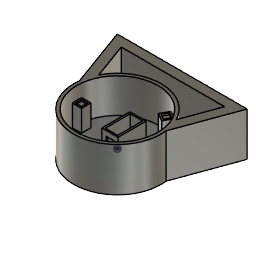
base (Autodesk Fusion 360 design; units mm, degrees)
part number: 2026-04-11-20-46-35-082
Autodesk Fusion 360 part; units mm, degrees
note: some values were not read from the file. Chosen so that the rebuilt part matches the saved one: which bodies a step acts on; that a step has no effect; which face or edge a step refers to. Set by a fixed rule: which sketch regions a step uses.
sketch "Esboço1" plane through (0, 0, 0) normal (0, 0, 1) x (1, 0, 0)
  circle A0 centre (0, 0) radius 70
  circle A1 centre (0, 0) radius 65
  dimension "d1" = 140
  dimension "d2" = 130
  constraint coincident A0.centre A1.centre
  measures "d1" diameter of A0
  measures "d2" diameter of A1
extrude "Extrusão1" add sketch "Esboço1" along normal blind 45 makes body 1
sketch "Esboço2" plane through (0, 0, 0) normal (0, 0, 1) x (1, 0, 0)
  circle A0 centre (0, 0) radius 70
  constraint coincident A0.centre origin
extrude "Extrusão2" add sketch "Esboço2" along normal blind 5 bodies 1
sketch "Esboço3" plane through (0, 0, 0) normal (0, 0, 1) x (1, 0, 0)
  line L0 (-9.5, 19.5) -> (9.5, 19.5)
  line L1 (9.5, 19.5) -> (9.5, -19.5)
  line L2 (9.5, -19.5) -> (-9.5, -19.5)
  line L3 (-9.5, -19.5) -> (-9.5, 19.5)
  line L4 (-9.75, -19.75) -> (9.75, -19.75)
  line L5 (9.75, -19.75) -> (9.75, 19.75)
  line L6 (9.75, 19.75) -> (-9.75, 19.75)
  line L7 (-9.75, 19.75) -> (-9.75, -19.75)
  circle A0 centre (0, 0) radius 70
  line L8 (0, 0) -> (9.5, 0)
  line L9 (0, 0) -> (0, -19.5)
  dimension "d7" = 19
  dimension "d8" = 39
  dimension "d9" = 19.5
  dimension "d10" = 39.5
  dimension "d15" = 9.5
  dimension "d16" = 19.5
  constraint horizontal L0
  constraint vertical L1
  constraint horizontal L2
  constraint vertical L3
  constraint horizontal L4
  constraint vertical L5
  constraint horizontal L6
  constraint vertical L7
  constraint coincident A0.centre L8.start
  constraint perpendicular L5 L8
  constraint perpendicular L8 L9
  constraint coincident L2 L9.end
  constraint coincident L1 L8.end
  measures "d7" distance of L0.start L0.end
  measures "d8" distance of L0.start L2.end
  measures "d9" distance of L4.start L4.end
  measures "d10" distance of L4.start L6.end
  measures "d15" distance of A0.centre L8.end
  measures "d16" distance of A0.centre L9.end
sketch "Esboço5" plane through (0, 0, 0) normal (0, 0, 1) x (1, 0, 0)
sketch "Esboço6" plane through (0, 0, 0) normal (0, 0, -1) x (1, 0, 0)
  circle A0 centre (0, 0) radius 70
  line L0 (-9.5, 19.5) -> (9.5, 19.5)
  line L1 (9.5, 19.5) -> (9.5, -19.5)
  line L2 (9.5, -19.5) -> (-9.5, -19.5)
  line L3 (-9.5, -19.5) -> (-9.5, 19.5)
  line L4 (-70, 0) -> (70, 0)
  line L5 (-12, 22) -> (12, 22)
  line L6 (12, 22) -> (12, -22)
  line L7 (12, -22) -> (-12, -22)
  line L8 (-12, -22) -> (-12, 22)
  dimension "d19" = 19
  dimension "d20" = 39
  dimension "d21" = 24
  dimension "d22" = 44
  constraint horizontal L0
  constraint vertical L1
  constraint horizontal L2
  constraint vertical L3
  constraint coincident A0 L4.start
  constraint coincident A0 L4.end
  constraint horizontal L5
  constraint vertical L6
  constraint horizontal L7
  constraint vertical L8
  measures "d19" distance of L0.start L0.end
  measures "d20" distance of L0.start L2.end
  measures "d21" distance of L5.start L5.end
  measures "d22" distance of L5.start L7.end
extrude "Extrusão4" add sketch "Esboço6" against normal blind 38 contours L1 L2 L3 L4 L6 L7 L8 | L0 L1 L3 L4 L5 L6 L8 bodies 1
move_body "Mover1" bodies 1 to x (1, 0, 0) y (0, 1, 0) z (0, 0, 1) at (0, 0, 10)
extrude "Extrusão5" add 1 faces at (2.4201, -10.6031, 10) along direction (0, 0, -1) blind 10 on bodies 1 bodies 1
sketch "Esboço7" plane through (0, 0, 15) normal (0, 0, 1) x (-1, 0, 0)
  circle A0 centre (0, 0) radius 65
  line L0 (-12, -22) -> (-12, 22)
  line L1 (-12, 22) -> (12, 22)
  line L2 (12, 22) -> (12, -22)
  line L3 (12, -22) -> (-12, -22)
  line L4 (-20, 30) -> (20, 30)
  line L5 (20, 30) -> (20, -30)
  line L6 (20, -30) -> (-20, -30)
  line L7 (-20, -30) -> (-20, 30)
  constraint horizontal L4
  constraint vertical L5
  constraint horizontal L6
  constraint vertical L7
extrude "Extrusão6" cut sketch "Esboço7" along normal blind 0.01 contours L0 L1 L2 L3 | L4 L5 L6 L7 bodies 1 makes body 2 at (69.913, -3.4892, 18.3333)
sketch "Esboço8" plane through (0, 0, 15) normal (0, 0, 1) x (-1, 0, 0)
  circle A0 centre (0, 0) radius 65
  circle A1 centre (0, 0) radius 2.5
  dimension "d29" = 5
  constraint coincident A0.centre A1.centre
  measures "d29" diameter of A1
move_body "Mover2" bodies 1 to x (1, 0, 0) y (0, 1, 0) z (0, 0, 1) at (0, 9, 0)
move_body "Mover3" bodies 1 to x (1, 0, 0) y (0, 1, 0) z (0, 0, 1) at (0, 1.5, 0)
move_body "Mover4" bodies 1 to x (1, 0, 0) y (0, 1, 0) z (0, 0, 1) at (0, 0, -0.02)
combine "Combinar1" operation add target body 2 tool bodies 1
fillet "Arredondamento1" radius 5 tangency weight 0.69913 4 edges at (-12, 10.5, 15) (0, -11.5, 15) (12, 10.5, 15) (0, 32.5, 15) on bodies 2
sketch "Esboço9" plane through (0, -11.5, 0) normal (0, -1, 0) x (1, 0, 0)
  line L0 (12, 20) -> (-12, 20)
  line L1 (12, 20) -> (12, 47.98)
  line L2 (12, 47.98) -> (-12, 47.98)
  line L3 (-12, 47.98) -> (-12, 20)
  line L4 (-4.8756, 37.7433) -> (5.1244, 37.7433)
  line L5 (5.1244, 37.7433) -> (5.1244, 22.7433)
  line L6 (5.1244, 22.7433) -> (-4.8756, 22.7433)
  line L7 (-4.8756, 22.7433) -> (-4.8756, 37.7433)
  dimension "d32" = 10
  dimension "d33" = 15
  constraint horizontal L4
  constraint vertical L5
  constraint horizontal L6
  constraint vertical L7
  measures "d32" distance of L4.start L4.end
  measures "d33" distance of L4.start L6.end
extrude "Extrusão7" add sketch "Esboço9" along normal blind 22 separate body contours L4 L5 L6 L7 makes body 3
move_body "Mover5" bodies 3 to x (1, 0, 0) y (0, 1, 0) z (0, 0, 1) at (0, 0, -7.743)
move_body "Mover6" bodies 3 to x (1, 0, 0) y (0, 1, 0) z (0, 0, 1) at (-0.124, 0, 0)
move_body "Mover7" bodies 3 to x (1, 0, 0) y (0, 1, 0) z (0, 0, 1) at (0, 60, 0)
combine "Combinar2" operation cut target body 2 tool bodies 3
extrude "Extrusão8" cut 1 faces at (-11.1667, 4, 47.98) along direction (0, 0, -1) blind 4.98 on bodies 2 bodies 2
sketch "Esboço10" plane through (0, 0, 15) normal (0, 0, 1) x (-1, 0, 0)
  line L0 (-32.5, 56.2917) -> (-26.0048, 60.0417)
  line L1 (-32.5, 56.2917) -> (-38.9952, 52.5417)
  line L2 (-38.9952, 52.5417) -> (-30.9952, 38.6852)
  line L3 (-26.0048, 60.0417) -> (-18.5048, 47.0513)
  line L4 (-18.5048, 47.0513) -> (-31.4952, 39.5513)
  line L5 (-32.5, -56.2917) -> (-38.9952, -52.5417)
  line L6 (-32.5, -56.2917) -> (-26.0048, -60.0417)
  line L7 (-38.9952, -52.5417) -> (-31.4952, -39.5513)
  line L8 (-26.0048, -60.0417) -> (-18.5048, -47.0513)
  line L9 (-31.4952, -39.5513) -> (-18.5048, -47.0513)
  line L10 (65, 0) -> (65, 7.5)
  line L11 (65, 0) -> (65, -7.5)
  line L12 (65, 7.5) -> (50, 7.5)
  line L13 (65, -7.5) -> (50, -7.5)
  line L14 (50, 7.5) -> (50, -7.5)
  line L15 (59.9632, 5) -> (62.5, 5)
  line L16 (52.5, 1) -> (52.5, -5)
  line L17 (52.5, 5) -> (52.5, 1)
  line L18 (52.5, -5) -> (62.5, -5)
  line L19 (62.5, 5) -> (62.5, -5)
  line L20 (52.5, 5) -> (62.5, 5)
  line L21 (-24.9107, -53.1467) -> (-26.9199, -56.6266)
  line L22 (-33.0801, -47.2965) -> (-30.5801, -42.9663)
  line L23 (-31.25, -54.1266) -> (-35.5801, -51.6266)
  line L24 (-24.9107, -53.1467) -> (-21.9199, -47.9663)
  line L25 (-35.5801, -51.6266) -> (-26.9199, -56.6266)
  line L26 (-35.5801, -51.6266) -> (-30.5801, -42.9663)
  line L27 (-30.5801, -42.9663) -> (-21.9199, -47.9663)
  line L28 (-21.9199, -47.9663) -> (-26.9199, -56.6266)
  line L29 (-31.25, 54.1266) -> (-35.5801, 51.6266)
  line L30 (-24.4199, 52.2965) -> (-26.9199, 56.6266)
  line L31 (-26.25, 45.4663) -> (-21.9199, 47.9663)
  line L32 (-30.5801, 42.9663) -> (-21.9199, 47.9663)
  line L33 (-21.9199, 47.9663) -> (-26.9199, 56.6266)
  line L34 (-26.9199, 56.6266) -> (-35.5801, 51.6266)
  line L35 (-35.5801, 51.6266) -> (-30.5801, 42.9663)
  dimension "d39" = 65
  dimension "d41" = 7.5
  dimension "d42" = 7.5
  dimension "d43" = 16
  dimension "d44" = 15
  dimension "d52" = 7.5
  dimension "d53" = 7.5
  dimension "d54" = 15
  dimension "d55" = 15
  dimension "d57" = 7.5
  dimension "d58" = 7.5
  dimension "d59" = 15
  dimension "d60" = 15
  dimension "d64" = 2.5
  dimension "d68" = 2.5
  constraint perpendicular L1 L2
  constraint perpendicular L0 L3
  constraint coincident L2 L4.end
  constraint perpendicular L2 L4
  constraint perpendicular L5 L7
  constraint perpendicular L6 L8
  constraint perpendicular L10 L12
  constraint perpendicular L11 L13
  constraint perpendicular L13 L14
  constraint perpendicular L18 L19
  constraint perpendicular L19 L20
  constraint perpendicular L21 L25
  measures "d39" distance of origin L0.start
  measures "d41" distance of L0.start L0.end
  measures "d42" distance of L0.start L1.end
  measures "d43" distance of L1.end L2.end
  measures "d44" distance of L0.end L3.end
  measures "d52" distance of L5.start L5.end
  measures "d53" distance of L5.start L6.end
  measures "d54" distance of L5.end L7.end
  measures "d55" distance of L6.end L8.end
  measures "d57" distance of L10.start L10.end
  measures "d58" distance of L10.start L11.end
  measures "d59" distance of L10.end L12.end
  measures "d60" distance of L11.end L13.end
  measures "d64" distance of L5.start L23.start
  measures "d68" distance of L0.start L29.start
extrude "Extrusão9" add sketch "Esboço10" along normal blind 45 contours L15 L16 L17 L18 L19 L20 | L21 L22 L23 L24 L25 L26 L27 L28 | L29 L30 L31 L32 L33 L34 L35 bodies 2
extrude "Extrusão10" add sketch "Esboço10" along normal blind 45 separate body makes body 4 at (34.6651, -55.0417, 45) makes body 5 at (30.3349, 57.5417, 45) makes body 6 at (-65, -2.5, 45)
extrude "Extrusão11" cut 3 faces at (-50.8333, 1.6667, 60) (35.3568, -47.9065, 60) (35.3568, 47.9065, 60) along direction (0, 0, -1) blind 5 on bodies 4 5 6 bodies 4 5 6
extrude "Extrusão12" cut 3 faces at (28.14, 52.0732, 60) (31.0267, -50.4065, 60) (-59.1667, 1.6667, 60) along direction (0, 0, -1) blind 7 on bodies 2 bodies 2
extrude "Extrusão13" add 1 faces at (68.0727, -3.4777, 55) along direction (0, 0, 1) blind 15 on bodies 2 bodies 2 4 5 6
sketch "Esboço11" plane through (0, 0, 0) normal (0, 0, 1) x (1, 0, 0)
  line L0 (-70, 10) -> (-104.202, 103.9693)
  line L1 (-70, 10) -> (30, 10) construction
  line L2 (-104.202, 103.9693) -> (104.202, 103.9693)
  line L3 (79.2766, 79.3444) -> (61.5837, 30.7335)
  line L4 (-77.6538, 74.8857) -> (-82.7798, 88.9693)
  line L5 (-77.6538, 74.8857) -> (-61.6137, 30.8159)
  line L6 (61.5837, 30.7335) -> (82.7798, 88.9693)
  line L7 (-82.7798, 88.9693) -> (82.7798, 88.9693)
  line L8 (70, 10) -> (69.2581, 7.9618)
  line L9 (69.2581, 7.9618) -> (61.5837, 30.7335)
  line L10 (69.2581, 7.9618) -> (104.202, 103.9693)
  line L11 (-70, 10) -> (-69.3383, 8.1819)
  line L12 (-69.3383, 8.1819) -> (-61.6137, 30.8159)
  line L13 (-61.6137, 30.8159) -> (61.5837, 30.7335)
  dimension "d82" = 110
  dimension "d83" = 100
  dimension "d85" = 100
  constraint horizontal L1
  constraint parallel L0 L11
  measures "d82" angle of L0 L1
  measures "d83" distance of L0.start L0.end
  measures "d85" distance of L8.start L2.end
extrude "Extrusão14" add sketch "Esboço11" along normal blind 15 contours L3 L4 L5 L6 L7 L13 bodies 2
extrude "Extrusão15" add sketch "Esboço11" along normal blind 70 contours L0 L2 L3 L4 L5 L6 L7 L8 L9 L10 L11 L12 bodies 2
extrude "Extrusão16" add 3 faces at (26.86, 43.1896, 55) (-50.8333, 1.6667, 55) (26.86, -43.1896, 55) along direction (0, 0, 1) blind 1 on bodies 2 bodies 2
extrude "Extrusão17" cut 3 faces at (-50.8333, 1.6667, 56) (26.86, -43.1896, 56) (26.86, 43.1896, 56) along direction (0, 0, -1) blind 0.5 on bodies 2 bodies 2
extrude "Extrusão18" cut 3 faces at (28.14, 52.0732, 53) (-59.1667, 1.6667, 53) (31.0267, -50.4065, 53) along direction (0, 0, -1) blind 10 on bodies 2 bodies 2
extrude "Extrusão19" add 3 faces at (28.14, 52.0732, 43) (-59.1667, 1.6667, 43) (31.0267, -50.4065, 43) along direction (0, 0, 1) blind 4 on bodies 2 bodies 2
extrude "Extrusão20" cut 3 faces at (-50.8333, 1.6667, 55.5) (26.86, 43.1896, 55.5) (26.86, -43.1896, 55.5) along direction (0, 0, -1) blind 9.5 on bodies 2 bodies 2
extrude "Extrusão21" add 3 faces at (-50.8333, 1.6667, 46) (26.86, 43.1896, 46) (26.86, -43.1896, 46) along direction (0, 0, 1) blind 3.5 on bodies 2 bodies 2
form "Forma1" [no effect]
extrude "Extrusão22" add 1 faces at (-4, -11.5, 27.6667) along direction (0, -1, 0) blind 0.5 on bodies 2 bodies 2
extrude "Extrusão23" add 1 faces at (-1.6665, 32.5, 38.6668) along direction (0, 1, 0) blind 0.5 on bodies 2 bodies 2
extrude "Extrusão24" cut 1 faces at (-3.1667, -9, 24.3333) along direction (0, -1, 0) blind 0.5 on bodies 2 bodies 2
extrude "Extrusão25" cut 1 faces at (-1.6665, 30, 38.6668) along direction (0, 1, 0) blind 0.5 on bodies 2 bodies 2
extrude "Extrusão26" cut 1 faces at (9.5, 3.8333, 24.3333) along direction (1, 0, 0) blind 0.5 on bodies 2 bodies 2
extrude "Extrusão27" cut 1 faces at (-9.5, 17.1667, 24.3333) along direction (-1, 0, 0) blind 0.5 on bodies 2 bodies 2
extrude "Extrusão28" add 1 faces at (12, 17.8333, 35.3333) along direction (1, 0, 0) blind 1 on bodies 2 bodies 2
extrude "Extrusão29" add 1 faces at (-12, 17.8333, 35.3333) along direction (-1, 0, 0) blind 1 on bodies 2 bodies 2
sketch "Esboço12" plane through (0, 0, 0) normal (0, 0, 1) x (1, 0, 0)
extrude "Extrusão30" add 1 faces at (-4.9996, 32, 26.6669) along direction (1, 0, 0) blind 11 on bodies 2 bodies 2
ref_plane "Plano de trabalho1" through (0, -9.5, 29) normal (0, 1, 0) x (0, 0, 1)
sketch "Esboço13" plane through (0, -9.5, 0) normal (0, 1, 0) x (1, 0, 0)
  line L0 (0, -15) -> (6, -15)
  line L1 (6, -15) -> (6, -35)
  line L2 (0, -15) -> (-6, -15)
  line L3 (-6, -15) -> (-6, -35)
  line L4 (-6, -35) -> (6, -35)
  constraint horizontal L0
  constraint perpendicular L0 L1
  constraint perpendicular L1 L2
  constraint perpendicular L0 L3
  constraint perpendicular L1 L4
extrude "Extrusão31" cut sketch "Esboço13" against normal blind 10 bodies 2
extrude "Extrusão3" [rolled back] along distance 29 taper angle 0
sketch "Esboço4" plane through (0, 0, 0) normal (0, 0, 1) x (1, 0, 0)
equation "d101 = 0.00 mm - 9.5 mm"
